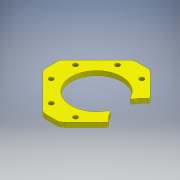
# Autodesk Inventor part: VAM_housing_top
Saved by Autodesk Inventor 2016 (Build 200138000, 138)
## iProperties
Created: 2015-12-08
Part Number: VAM_housing_top
Material: Generic
Document SubType Name: Modeling
Designer: lk8187
Density: 1 g/cm^3
Appearance: Smooth - Yellow
Author: lk8187
Autodesk Inventor part; units mm, degrees
ref_plane "YZ Plane" through (0, 0, 0) normal (1, 0, 0) x (0, 1, 0)
ref_plane "XZ Plane" through (0, 0, 0) normal (0, 1, 0) x (-1, 0, 0)
ref_plane "XY Plane" through (0, 0, 0) normal (0, 0, 1) x (1, 0, 0)
sketch "Sketch1" plane through (0, 0, 0) normal (0, 0, 1) x (1, 0, 0)
  arc A0 (-3.5858, 30.4056) -> (-7.1213, 28.9411) centre (-3.5858, 25.4056) ccw
  line L0 (-7.1213, 28.9411) -> (-28.9411, 7.1213)
  arc A1 (-28.9411, 7.1213) -> (-30.4056, 3.5858) centre (-25.4056, 3.5858) ccw
  line L1 (-30.4056, 3.5858) -> (-30.4056, -3.5858)
  arc A2 (-30.4056, -3.5858) -> (-28.9411, -7.1213) centre (-25.4056, -3.5858) ccw
  line L2 (-28.9411, -7.1213) -> (-7.1213, -28.9411)
  arc A3 (-7.1213, -28.9411) -> (-3.5858, -30.4056) centre (-3.5858, -25.4056) ccw
  line L3 (-3.5858, -30.4056) -> (3.5858, -30.4056)
  arc A4 (3.5858, -30.4056) -> (7.1213, -28.9411) centre (3.5858, -25.4056) ccw
  line L4 (7.1213, -28.9411) -> (22.1833, -13.8792)
  arc A5 (16, -5.7446) -> (22.1833, -13.8792) centre (32, 0) ccw
  arc A6 (16, 5.7446) -> (16, -5.7446) centre (0, 0) ccw
  arc A7 (22.1833, 13.8792) -> (16, 5.7446) centre (32, 0) ccw
  line L5 (22.1833, 13.8792) -> (7.1213, 28.9411)
  arc A8 (7.1213, 28.9411) -> (3.5858, 30.4056) centre (3.5858, 25.4056) ccw
  line L6 (3.5858, 30.4056) -> (-3.5858, 30.4056)
  circle A9 centre (-8.1317, 22.2739) radius 1.5
  circle A10 centre (-22.2739, 8.1317) radius 1.5
  circle A11 centre (8.1317, -22.2739) radius 1.5
  circle A12 centre (-8.1317, -22.2739) radius 1.5
  circle A13 centre (8.1317, 22.2739) radius 1.5
  circle A14 centre (-22.2739, -8.1317) radius 1.5
  point P0 (0, 0)
  constraints: 18 point on circle, 15 centre point, 14 end point, 2 horizontal, 1 vertical, 50 other
extrude "Extrusion1" add sketch "Sketch1" along normal blind 3
fillet "Fillet1" radius 1 4 edges at (16, 5.7446, 1.5) (22.1833, 13.8792, 1.5) (16, -5.7446, 1.5) (22.1833, -13.8792, 1.5)
body "Solid1"
